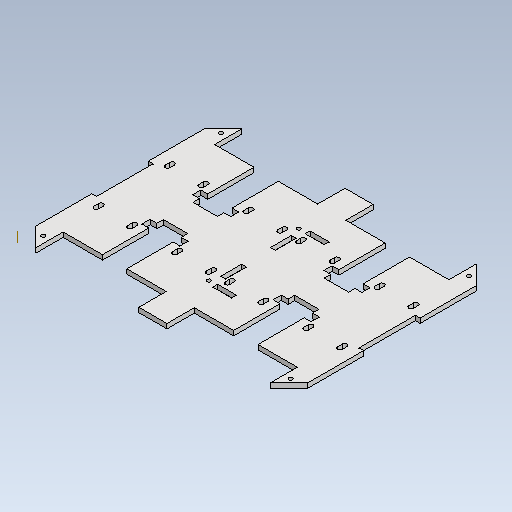
# Autodesk Inventor part: floor
Saved by Autodesk Inventor 2025 (Build 290162000, 162)
## iProperties
Created: 2025-08-20
Part Number: floor
Material: Generic
Document SubType Name: Modeling
Designer: HP
Density: 1 g/cm^3
Appearance: Default
Author: HP
Autodesk Inventor part; units mm, degrees
ref_plane "YZ Plane" through (0, 0, 0) normal (1, 0, 0) x (0, 1, 0)
ref_plane "XZ Plane" through (0, 0, 0) normal (0, 1, 0) x (-1, 0, 0)
ref_plane "XY Plane" through (0, 0, 0) normal (0, 0, 1) x (1, 0, 0)
sketch "Sketch1" plane through (0, 0, 0) normal (0, 1, 0) x (-1, 0, 0)
  line L0 (145, 110) -> (-145, 110)
  line L1 (-145, 110) -> (-145, -110)
  line L2 (-145, -110) -> (145, -110)
  line L3 (145, -110) -> (145, 110)
  line L4 (145, 110) -> (-145, -110) construction
  line L5 (-145, 110) -> (145, -110) construction
  line L6 (125, -80.8333) -> (15, -80.8333)
  line L7 (15, -80.8333) -> (15, -115.8333)
  line L8 (15, -115.8333) -> (125, -115.8333)
  line L9 (125, -115.8333) -> (125, -80.8333)
  line L10 (125, -80.8333) -> (15, -115.8333) construction
  line L11 (15, -80.8333) -> (125, -115.8333) construction
  line L12 (-15, -115.8333) -> (-125, -115.8333)
  line L13 (-125, -115.8333) -> (-125, -80.8333)
  line L14 (-125, -80.8333) -> (-15, -80.8333)
  line L15 (-15, -80.8333) -> (-15, -115.8333)
  line L16 (-15, -115.8333) -> (-125, -80.8333) construction
  line L17 (-125, -115.8333) -> (-15, -80.8333) construction
  line L18 (0, 110) -> (0, -110) construction
  point P0 (0, 0)
  point P1 (70, -98.3333)
  point P2 (-70, -98.3333)
  point P3 (0, 0)
  point P4 (-125, -110)
  point P5 (-15, -110)
  dimension "d1" = 110
  dimension "d2" = 110
  dimension "d3" = 35
  dimension "d4" = 35
  dimension "d5" = 140
  dimension "d6" = 11.6667
  dimension "d7" = 220
  dimension "d8" = 290
  constraints: 38 end point, 8 midpoint, 6 parallel, 3 horizontal, 3 perpendicular, 1 coincident, 1 horizontal alignment, 1 other
  measures "d1" distance between parallel lines of L7 L9
  measures "d2" distance between parallel lines of L13 L15
  measures "d3" distance between parallel lines of L6 L8
  measures "d4" distance between parallel lines of L14 L12
  measures "d5" distance of point (-70, -98.333) point (70, -98.333)
  measures "d6" distance from line of L2 point (70, -98.333)
  measures "d7" distance between parallel lines of L0 L2
  measures "d8" distance between parallel lines of L1 L3
extrude "Extrusion1" add sketch "Sketch1" along normal blind 5 contours L3 L2 L9 L6 L7 L15 L14 L13 L1 L0 | L2 L7 L6 L9 | L13 L14 L15 L2
extrude "Extrusion2" cut sketch "Sketch1" along normal blind 5 contours L9 L8 L7 L2 | L2 L7 L6 L9 | L13 L14 L15 L2
mirror "Mirror1" about plane through (0, 0, 0) normal (0, 0, 1) of "Extrusion2"
sketch "Sketch2" plane through (0, 5, 0) normal (0, 1, 0) x (1, 0, 0)
  line L0 (-125, -110) -> (-125, -80.8333) projected
  line L1 (-125, -80.8333) -> (-15, -80.8333) projected
  line L2 (-15, -80.8333) -> (-15, -110) projected
  line L3 (-15, -110) -> (15, -110) projected
  line L4 (15, -110) -> (15, -80.8333) projected
  line L5 (15, -80.8333) -> (125, -80.8333) projected
  line L6 (125, -80.8333) -> (125, -110) projected
  line L7 (125, -110) -> (145, -110) projected
  line L8 (145, -110) -> (145, 110) projected
  line L9 (145, 110) -> (125, 110) projected
  line L10 (125, 110) -> (125, 80.8333) projected
  line L11 (125, 80.8333) -> (15, 80.8333) projected
  line L12 (15, 80.8333) -> (15, 110) projected
  line L13 (15, 110) -> (-15, 110) projected
  line L14 (-15, 110) -> (-15, 80.8333) projected
  line L15 (-15, 80.8333) -> (-125, 80.8333) projected
  line L16 (-125, 80.8333) -> (-125, 110) projected
  line L17 (-125, 110) -> (-145, 110) projected
  line L18 (-145, 110) -> (-145, -110) projected
  line L19 (-145, -110) -> (-125, -110) projected
  line L20 (83, 80.8333) -> (57, 80.8333)
  line L21 (57, 80.8333) -> (57, 15.8333)
  line L22 (57, 15.8333) -> (83, 15.8333)
  line L23 (83, 15.8333) -> (83, 80.8333)
  line L24 (83, 80.8333) -> (57, 15.8333) construction
  line L25 (57, 80.8333) -> (83, 15.8333) construction
  line L26 (49.68, 22.7333) -> (57, 22.7333)
  line L27 (57, 22.7333) -> (57, 31.4333)
  line L28 (57, 31.4333) -> (49.68, 31.4333)
  line L29 (49.68, 31.4333) -> (49.68, 22.7333)
  line L30 (49.68, 22.7333) -> (57, 31.4333) construction
  line L31 (57, 22.7333) -> (49.68, 31.4333) construction
  line L32 (83, 22.7333) -> (90.32, 22.7333)
  line L33 (90.32, 22.7333) -> (90.32, 31.4333)
  line L34 (90.32, 31.4333) -> (83, 31.4333)
  line L35 (83, 31.4333) -> (83, 22.7333)
  line L36 (83, 22.7333) -> (90.32, 31.4333) construction
  line L37 (90.32, 22.7333) -> (83, 31.4333) construction
  point P0 (0, 0)
  point P1 (70, 48.3333)
  point P2 (70, 80.8333)
  point P3 (53.34, 27.0833)
  point P4 (86.66, 27.0833)
  dimension "d14" = 26
  dimension "d15" = 65
  dimension "d79" = 7.32
  dimension "d80" = 8.7
  dimension "d81" = 11.25
  dimension "d82" = 8.7
  dimension "d83" = 7.32
  constraints: 36 end point, 7 midpoint, 6 parallel, 3 collinear, 3 horizontal, 3 perpendicular, 1 horizontal alignment, 1 vertical alignment
  measures "d14" distance between parallel lines of L23 L21
  measures "d15" distance between parallel lines of L20 L22
  measures "d79" distance between parallel lines of L27 L29
  measures "d80" distance between parallel lines of L26 L28
  measures "d81" distance from line of L22 point (53.34, 27.083)
  measures "d82" distance between parallel lines of L32 L34
  measures "d83" distance between parallel lines of L33 L35
extrude "Extrusion3" cut sketch "Sketch2" against normal through all contours L11 L23 L22 L21 | L21 L26 L29 L28 | L34 L33 L32 L23
mirror "Mirror2" about plane through (0, 0, 0) normal (0, 0, 1) of "Extrusion3"
mirror "Mirror3" about plane through (0, 0, 0) normal (1, 0, 0) of "Extrusion3", "Mirror2"
chamfer "Chamfer1" distance 20 angle 45 4 edges at (145, 2.5, 110) (145, 2.5, -110) (-145, 2.5, -110) (-145, 2.5, 110)
sketch "Sketch3" plane through (0, 5, 0) normal (0, 1, 0) x (1, 0, 0)
  line L0 (-125, -110) -> (-145, -90) construction
  line L1 (-125, -110) -> (-125, -80.8333) construction
  line L2 (-125, -80.8333) -> (-83, -80.8333) construction
  line L3 (-83, -80.8333) -> (-83, -31.4333) construction
  line L4 (-83, -15.8333) -> (-57, -15.8333) construction
  line L5 (-57, -15.8333) -> (-57, -22.7333) construction
  line L6 (-57, -80.8333) -> (-15, -80.8333) construction
  line L7 (-15, -80.8333) -> (-15, -110) construction
  line L8 (-15, -110) -> (15, -110) construction
  line L9 (15, -110) -> (15, -80.8333) construction
  line L10 (15, -80.8333) -> (57, -80.8333) construction
  line L11 (57, -80.8333) -> (57, -31.4333) construction
  line L12 (57, -15.8333) -> (83, -15.8333) construction
  line L13 (83, -31.4333) -> (83, -80.8333) construction
  line L14 (83, -80.8333) -> (125, -80.8333) construction
  line L15 (125, -80.8333) -> (125, -110) construction
  line L16 (145, -90) -> (125, -110) construction
  line L17 (145, -90) -> (145, 90) construction
  line L18 (125, 110) -> (145, 90) construction
  line L19 (125, 110) -> (125, 80.8333) construction
  line L20 (125, 80.8333) -> (83, 80.8333) construction
  line L21 (83, 80.8333) -> (83, 31.4333) construction
  line L22 (83, 15.8333) -> (57, 15.8333) construction
  line L23 (57, 31.4333) -> (57, 80.8333) construction
  line L24 (57, 80.8333) -> (15, 80.8333) construction
  line L25 (15, 80.8333) -> (15, 110) construction
  line L26 (15, 110) -> (-15, 110) construction
  line L27 (-15, 110) -> (-15, 80.8333) construction
  line L28 (-15, 80.8333) -> (-57, 80.8333) construction
  line L29 (-57, 80.8333) -> (-57, 31.4333) construction
  line L30 (-57, 15.8333) -> (-83, 15.8333) construction
  line L31 (-83, 15.8333) -> (-83, 22.7333) construction
  line L32 (-83, 80.8333) -> (-125, 80.8333) construction
  line L33 (-125, 80.8333) -> (-125, 110) construction
  line L34 (-145, 90) -> (-125, 110) construction
  line L35 (-145, 90) -> (-145, -90) construction
  line L36 (-140, 30.1) -> (-145, 30.1)
  line L37 (-145, 30.1) -> (-145, -30.1)
  line L38 (-145, -30.1) -> (-140, -30.1)
  line L39 (-140, -30.1) -> (-140, 30.1)
  line L40 (-140, 30.1) -> (-145, -30.1) construction
  line L41 (-145, 30.1) -> (-140, -30.1) construction
  line L42 (145, -30.1) -> (140, -30.1)
  line L43 (140, -30.1) -> (140, 30.1)
  line L44 (140, 30.1) -> (145, 30.1)
  line L45 (145, 30.1) -> (145, -30.1)
  line L46 (145, -30.1) -> (140, 30.1) construction
  line L47 (140, -30.1) -> (145, 30.1) construction
  line L48 (145, -90) -> (145, 90) projected
  line L49 (-145, 90) -> (-145, -90) projected
  circle A0 centre (-132, -95) radius 2.1
  circle A1 centre (132, -95) radius 2.1
  circle A2 centre (-2.4, -48) radius 2.1
  line L50 (-130, -35.5) -> (-130, -40.5) construction
  line L51 (-132.5, -35.5) -> (-132.5, -40.5)
  line L52 (-127.5, -40.5) -> (-127.5, -35.5)
  arc A3 (-127.5, -35.5) -> (-132.5, -35.5) centre (-130, -35.5) ccw
  arc A4 (-132.5, -40.5) -> (-127.5, -40.5) centre (-130, -40.5) ccw
  line L53 (-94, -35.5) -> (-94, -40.5) construction
  line L54 (-96.5, -35.5) -> (-96.5, -40.5)
  line L55 (-91.5, -40.5) -> (-91.5, -35.5)
  arc A5 (-91.5, -35.5) -> (-96.5, -35.5) centre (-94, -35.5) ccw
  arc A6 (-96.5, -40.5) -> (-91.5, -40.5) centre (-94, -40.5) ccw
  line L56 (-46, -35.5) -> (-46, -40.5) construction
  line L57 (-48.5, -35.5) -> (-48.5, -40.5)
  line L58 (-43.5, -40.5) -> (-43.5, -35.5)
  arc A7 (-43.5, -35.5) -> (-48.5, -35.5) centre (-46, -35.5) ccw
  arc A8 (-48.5, -40.5) -> (-43.5, -40.5) centre (-46, -40.5) ccw
  arc A9 (-7.5, -35.5) -> (-12.5, -35.5) centre (-10, -35.5) ccw
  line L59 (-10, -35.5) -> (-10, -40.5) construction
  line L60 (-12.5, -35.5) -> (-12.5, -40.5)
  line L61 (-7.5, -40.5) -> (-7.5, -35.5)
  arc A10 (-12.5, -40.5) -> (-7.5, -40.5) centre (-10, -40.5) ccw
  line L62 (10, -35.5) -> (10, -40.5) construction
  line L63 (7.5, -35.5) -> (7.5, -40.5)
  line L64 (12.5, -40.5) -> (12.5, -35.5)
  arc A11 (12.5, -35.5) -> (7.5, -35.5) centre (10, -35.5) ccw
  arc A12 (7.5, -40.5) -> (12.5, -40.5) centre (10, -40.5) ccw
  arc A13 (48.5, -35.5) -> (43.5, -35.5) centre (46, -35.5) ccw
  line L65 (46, -35.5) -> (46, -40.5) construction
  line L66 (43.5, -35.5) -> (43.5, -40.5)
  line L67 (48.5, -40.5) -> (48.5, -35.5)
  arc A14 (43.5, -40.5) -> (48.5, -40.5) centre (46, -40.5) ccw
  line L68 (94, -35.5) -> (94, -40.5) construction
  line L69 (91.5, -35.5) -> (91.5, -40.5)
  line L70 (96.5, -40.5) -> (96.5, -35.5)
  arc A15 (96.5, -35.5) -> (91.5, -35.5) centre (94, -35.5) ccw
  arc A16 (91.5, -40.5) -> (96.5, -40.5) centre (94, -40.5) ccw
  arc A17 (132.5, -35.5) -> (127.5, -35.5) centre (130, -35.5) ccw
  line L71 (130, -35.5) -> (130, -40.5) construction
  line L72 (127.5, -35.5) -> (127.5, -40.5)
  line L73 (132.5, -40.5) -> (132.5, -35.5)
  arc A18 (127.5, -40.5) -> (132.5, -40.5) centre (130, -40.5) ccw
  line L74 (0, -15.5) -> (5.2, -15.5)
  line L75 (5.2, -15.5) -> (5.2, -37.7)
  line L76 (5.2, -37.7) -> (0, -37.7)
  line L77 (0, -37.7) -> (0, -15.5)
  line L78 (0, -15.5) -> (5.2, -37.7) construction
  line L79 (5.2, -15.5) -> (0, -37.7) construction
  line L80 (5.8, -46.7333) -> (26, -46.7333)
  line L81 (26, -46.7333) -> (26, -51.9333)
  line L82 (26, -51.9333) -> (5.8, -51.9333)
  line L83 (5.8, -51.9333) -> (5.8, -46.7333)
  line L84 (5.8, -46.7333) -> (26, -51.9333) construction
  line L85 (26, -46.7333) -> (5.8, -51.9333) construction
  line L86 (-83, -31.4333) -> (-90.32, -31.4333) projected
  line L87 (-90.32, -31.4333) -> (-90.32, -22.7333) projected
  line L88 (-90.32, -22.7333) -> (-83, -22.7333) projected
  line L89 (-83, -22.7333) -> (-83, -15.8333) projected
  line L90 (-57, -22.7333) -> (-49.68, -22.7333) projected
  line L91 (-49.68, -22.7333) -> (-49.68, -31.4333) projected
  line L92 (-49.68, -31.4333) -> (-57, -31.4333) projected
  line L93 (-57, -31.4333) -> (-57, -80.8333) projected
  line L94 (57, -31.4333) -> (49.68, -31.4333) projected
  line L95 (49.68, -31.4333) -> (49.68, -22.7333) projected
  line L96 (49.68, -22.7333) -> (57, -22.7333) projected
  line L97 (57, -22.7333) -> (57, -15.8333) projected
  line L98 (83, -15.8333) -> (83, -22.7333) projected
  line L99 (83, -22.7333) -> (90.32, -22.7333) projected
  line L100 (90.32, -22.7333) -> (90.32, -31.4333) projected
  line L101 (90.32, -31.4333) -> (83, -31.4333) projected
  line L102 (83, 31.4333) -> (90.32, 31.4333) projected
  line L103 (90.32, 31.4333) -> (90.32, 22.7333) projected
  line L104 (90.32, 22.7333) -> (83, 22.7333) projected
  line L105 (83, 22.7333) -> (83, 15.8333) projected
  line L106 (57, 15.8333) -> (57, 22.7333) projected
  line L107 (57, 22.7333) -> (49.68, 22.7333) projected
  line L108 (49.68, 22.7333) -> (49.68, 31.4333) projected
  line L109 (49.68, 31.4333) -> (57, 31.4333) projected
  line L110 (-57, 31.4333) -> (-49.68, 31.4333) projected
  line L111 (-49.68, 31.4333) -> (-49.68, 22.7333) projected
  line L112 (-49.68, 22.7333) -> (-57, 22.7333) projected
  line L113 (-57, 22.7333) -> (-57, 15.8333) projected
  line L114 (-83, 22.7333) -> (-90.32, 22.7333) projected
  line L115 (-90.32, 22.7333) -> (-90.32, 31.4333) projected
  line L116 (-90.32, 31.4333) -> (-83, 31.4333) projected
  line L117 (-83, 31.4333) -> (-83, 80.8333) projected
  point P0 (0, 0)
  point P1 (-142.5, 0)
  point P2 (142.5, 0)
  point P3 (-145, 0)
  point P4 (145, 0)
  point P5 (-130, -38)
  point P6 (-145, 0)
  point P7 (-94, -38)
  point P8 (-46, -38)
  point P9 (-10, -38)
  point P10 (10, -38)
  point P11 (46, -38)
  point P12 (94, -38)
  point P13 (130, -38)
  point P14 (2.6, -26.6)
  point P15 (15.9, -49.3333)
  dimension "d21" = 5
  dimension "d22" = 60.2
  dimension "d23" = 5
  dimension "d24" = 60.2
  dimension "d27" = 4.2
  dimension "d28" = 13
  dimension "d29" = 5
  dimension "d30" = 4.2
  dimension "d31" = 5
  dimension "d32" = 13
  dimension "d38" = 4.2
  dimension "d39" = 142.6
  dimension "d41" = 5
  dimension "d42" = 5
  dimension "d43" = 15
  dimension "d45" = 38
  dimension "d46" = 5
  dimension "d47" = 5
  dimension "d48" = 36
  dimension "d49" = 5
  dimension "d50" = 5
  dimension "d51" = 5
  dimension "d52" = 5
  dimension "d53" = 36
  dimension "d54" = 5
  dimension "d55" = 5
  dimension "d56" = 5
  dimension "d57" = 5
  dimension "d58" = 36
  dimension "d59" = 5
  dimension "d60" = 5
  dimension "d61" = 5
  dimension "d62" = 5
  dimension "d63" = 36
  dimension "d64" = 8.5
  dimension "d65" = 8.5
  dimension "d66" = 8.5
  dimension "d67" = 8.5
  dimension "d69" = 5.2
  dimension "d70" = 22.2
  dimension "d73" = 5.2
  dimension "d74" = 20.2
  dimension "d75" = 31.5
  dimension "d76" = 129.1
  dimension "d77" = 142.4
  dimension "d78" = 26.6
  dimension "d84" = 48
  constraints: 112 end point, 32 point on circle, 32 tangent, 19 centre point, 19 midpoint, 16 parallel, 9 horizontal alignment, 8 vertical, 4 horizontal, 4 perpendicular, 2 collinear
  measures "d21" distance of L38.end L37.end
  measures "d22" distance of L37.end L36.end
  measures "d23" distance of L43.end L44.end
  measures "d24" distance between parallel lines of L42 L44
  measures "d27" diameter of A0
  measures "d28" distance from line of L49 A0.centre
  measures "d29" vertical distance of A0.centre L0.end
  measures "d30" diameter of A1
  measures "d31" vertical distance of L16.start A1.centre
  measures "d32" distance from line of L17 A1.centre
  measures "d38" diameter of A2
  measures "d39" distance from line of A2.centre L35
  measures "d41" distance of L50.start L50.end
  measures "d42" distance between parallel lines of L52 L51
  measures "d43" distance between parallel lines of L50 L35
  measures "d45" vertical distance of point (-130, -38) point (-142.5, 0)
  measures "d46" distance of L53.start L53.end
  measures "d47" distance between parallel lines of L55 L54
  measures "d48" distance of point (-94, -38) point (-130, -38)
  measures "d49" distance of L56.start L56.end
  measures "d50" distance between parallel lines of L58 L57
  measures "d51" distance of L59.start L59.end
  measures "d52" distance between parallel lines of L61 L60
  measures "d53" distance of point (-10, -38) point (-46, -38)
  measures "d54" distance of L62.start L62.end
  measures "d55" distance between parallel lines of L64 L63
  measures "d56" distance of L65.start L65.end
  measures "d57" distance between parallel lines of L67 L66
  measures "d58" distance of point (46, -38) point (10, -38)
  measures "d59" distance of L68.start L68.end
  measures "d60" distance between parallel lines of L70 L69
  measures "d61" distance of L71.start L71.end
  measures "d62" distance between parallel lines of L73 L72
  measures "d63" distance of point (130, -38) point (94, -38)
  measures "d64" distance between parallel lines of L3 L55
  measures "d65" distance between parallel lines of L5 L57
  measures "d66" distance between parallel lines of L11 L67
  measures "d67" distance between parallel lines of L69 L13
  measures "d69" distance between parallel lines of L75 L77
  measures "d70" distance between parallel lines of L76 L74
  measures "d73" distance between parallel lines of L82 L80
  measures "d74" distance between parallel lines of L81 L83
  measures "d75" distance from line of L6 point (15.9, -49.333)
  measures "d76" distance from line of L17 point (15.9, -49.333)
  measures "d77" distance from line of L17 point (2.6, -26.6)
  measures "d78" vertical distance of point (2.6, -26.6) point (0, 0)
  measures "d84" vertical distance of point (0, 0) A2.centre
extrude "Extrusion4" cut sketch "Sketch3" against normal through all contours L39 L38 L37 L36 | L42 L43 L44 L45
extrude "Extrusion5" cut sketch "Sketch3" against normal through all contours A0 | A1 | A2 | A3 L52 A4 L51 | A5 L55 A6 L54 | A7 L58 A8 L57 | L61 A10 L60 A9 | A11 L64 A12 L63 | L67 A14 L66 A13 | A15 L70 A16 L69 | L73 A18 L72 A17 | L74 L75 L76 L77 | L80 L81 L82 L83
mirror "Mirror4" about plane through (0, 0, 0) normal (0, 0, 1) of "Extrusion5"
equation "\"d2\" = d1"
equation "\"d4\" = d3"
equation "\"d6\" = 0.333333 * d3"
equation "\"d82\" = d80"
equation "\"d83\" = d79"
equation "\"d24\" = d22"
equation "\"d30\" = d27"
equation "\"d31\" = d29"
equation "\"d32\" = d28"
equation "\"d65\" = d64"
equation "\"d66\" = d65"
equation "\"d67\" = d64"
body "Solid1"
